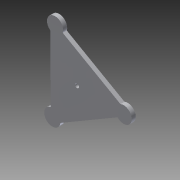
# Autodesk Inventor part: motorPlate
Saved by Autodesk Inventor 2013 (Build 170138000, 138)
## iProperties
Created: 2013-01-08
Part Number: motorPlate
Material: Aluminum 6061
Document SubType Name: Modeling
Designer: Nano
Density: 2.71 g/cm^3
Mass: 168.323 g
Surface Area: 225.935 cm^2
Volume: 62.1116 cm^3
Author: Nano
Autodesk Inventor part; units mm, degrees
ref_plane "YZ Plane" through (0, 0, 0) normal (1, 0, 0) x (0, 1, 0)
ref_plane "XZ Plane" through (0, 0, 0) normal (0, 1, 0) x (-1, 0, 0)
ref_plane "XY Plane" through (0, 0, 0) normal (0, 0, 1) x (1, 0, 0)
sketch "Sketch1" plane through (0, 0, 0) normal (0, 0, 1) x (1, 0, 0)
  circle A0 centre (-13.8429, -18.2704) radius 12.7 projected
  circle A1 centre (93.4781, -85.2045) radius 12.7 projected
  circle A2 centre (-18.149, -144.6801) radius 12.7 projected
  line L0 (103.5984, -82.1974) -> (-21.5072, -11.0096)
  line L1 (-21.5072, -11.0096) -> (-20.6049, -154.9481)
  line L2 (-20.6049, -154.9481) -> (103.5984, -82.1974)
  point P0 (0, 0)
  point P1 (-21.3977, -28.479)
  point P2 (-1.7779, -22.236)
  point P3 (88.4146, -73.5575)
  point P4 (84.0113, -93.6703)
  point P5 (-20.7472, -132.2488)
  point P6 (-5.5307, -146.1185)
  constraints: 6 end point, 6 point on circle, 6 point on line
extrude "Extrusion1" add sketch "Sketch1" along normal blind 6.35
sketch "Sketch2" plane through (0, 0, 6.35) normal (0, 0, 1) x (1, 0, 0)
  line L0 (-5.5307, -146.1185) -> (84.0113, -93.6703) projected
  line L1 (88.4146, -73.5575) -> (-1.7779, -22.236) projected
  line L2 (-21.3977, -28.479) -> (-20.7472, -132.2488) projected
  line L3 (43.3184, -47.8967) -> (11.3485, -104.0805) construction
  line L4 (39.2403, -119.8944) -> (11.3485, -72.2762) construction
  line L5 (-21.0724, -80.3639) -> (51.2351, -79.9106) construction
  line L6 (20.479, -80.1034) -> (20.5282, -87.9482) construction
  line L7 (15.9498, -80.1318) -> (22.7682, -84.0116) construction
  line L8 (25.0082, -80.075) -> (18.239, -84.04) construction
  circle A0 centre (20.4954, -82.7183) radius 3.175
  point P0 (0, 0)
  dimension "d2" = 6.35
  constraints: 12 end point, 11 point on line, 6 perpendicular, 3 midpoint, 1 centre point, 1 coincident
  measures "d2" diameter of A0
extrude "Extrusion2" cut sketch "Sketch2" against normal through all
body "Solid1"
